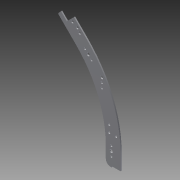
# Autodesk Inventor part: V5 Shooter Conveyor Plate P1 (45 Deg)
Saved by Autodesk Inventor 2014 SP1 (Build 180222100, 222)
## iProperties
Created: 2012-03-12
Part Number: V5 Shooter Conveyor Plate P1 (45 Deg)
Material: Aluminum-6061
Document SubType Name: Modeling
Designer: Moses
Mass: 110.618 g
Surface Area: 291.597 cm^2
Volume: 40.8185 cm^3
Density: 2.71 g/cm^3
Appearance: Aluminum - Flat
Author: Moses
Autodesk Inventor part; units mm, degrees
ref_plane "YZ Plane" through (0, 0, 0) normal (1, 0, 0) x (0, 1, 0)
ref_plane "XZ Plane" through (0, 0, 0) normal (0, 1, 0) x (-1, 0, 0)
ref_plane "XY Plane" through (0, 0, 0) normal (0, 0, 1) x (1, 0, 0)
sketch "Sketch1" plane through (0, 0, 0) normal (0, 0, 1) x (1, 0, 0)
  arc A0 (-15.749, 9.525) -> (-3.049, -3.175) centre (-3.049, 9.525) ccw
  line L0 (-3.049, -3.175) -> (0, -3.175)
  line L1 (0, -3.175) -> (0, 0)
  line L2 (0, 0) -> (24.5753, 0)
  line L3 (24.5753, 0) -> (24.5753, 41.4619)
  arc A1 (24.5753, 41.4619) -> (-69.0697, 267.5412) centre (-295.149, 41.4619) ccw
  line L4 (-69.0697, 267.5412) -> (-102.8779, 301.3493)
  line L5 (-102.8779, 301.3493) -> (-122.4112, 281.816)
  line L6 (-122.4112, 281.816) -> (-138.1267, 297.5314)
  line L7 (-138.1267, 297.5314) -> (-144.8619, 290.7962)
  arc A2 (-144.8619, 290.7962) -> (-144.8619, 286.3061) centre (-142.6168, 288.5511) ccw
  line L8 (-144.8619, 286.3061) -> (-97.5834, 239.0276)
  arc A3 (-15.749, 41.4619) -> (-97.5834, 239.0276) centre (-295.149, 41.4619) ccw
  line L9 (-15.749, 41.4619) -> (-15.749, 9.525)
  circle A4 centre (-1.0086, 22.225) radius 2.8448
  circle A5 centre (-1.0086, 47.625) radius 2.8448
  circle A6 centre (-26.9212, 171.2375) radius 2.85
  circle A7 centre (-26.9212, 183.9375) radius 2.85
  circle A8 centre (-26.9212, 196.6375) radius 4
  circle A9 centre (-73.0746, 241.3501) radius 2.85
  circle A10 centre (-55.1141, 223.3895) radius 2.85
  circle A11 centre (-7.1747, 76.2) radius 3.3782
  circle A12 centre (11.8753, 76.2) radius 3.3782
  circle A13 centre (-7.1747, 95.25) radius 3.3782
  circle A14 centre (-107.368, 287.8789) radius 3.3782
  circle A15 centre (-94.108, 280.5097) radius 3.3782
  circle A16 centre (-87.758, 270.9847) radius 3.3782
  circle A17 centre (-1.0086, 34.925) radius 4.15
  circle A18 centre (-64.0943, 232.3698) radius 4.15
  line L10 (-97.5834, 239.0276) -> (-69.0697, 267.5412) construction
  line L11 (-15.749, 41.4619) -> (24.5753, 41.4619) construction
  line L12 (-1.0086, 47.625) -> (-1.0086, 22.225) construction
  line L13 (-7.1747, 76.2) -> (11.8753, 76.2) construction
  line L14 (-7.1747, 76.2) -> (-7.1747, 95.25) construction
  line L15 (-26.9212, 196.6375) -> (-26.9212, 171.2375) construction
  line L16 (-73.0746, 241.3501) -> (-55.1141, 223.3895) construction
  dimension "d0" = 279.4
  dimension "d1" = 319.7243
  dimension "d2" = 6.7564
  dimension "d3" = 6.7564
  dimension "d4" = 6.7564
  dimension "d5" = 5.7
  dimension "d6" = 8.3
  dimension "d7" = 5.7
  dimension "d8" = 8
  dimension "d9" = 5.7
  dimension "d10" = 5.7
  dimension "d11" = 3.175
  dimension "d12" = 12.7
  dimension "d13" = 22.225
  dimension "d14" = 27.6243
  dimension "d15" = 47.8119
  dimension "d16" = 70.0369
  dimension "d17" = 66.8619
  dimension "d18" = 45
  dimension "d19" = 6.7564
  dimension "d20" = 6.7564
  dimension "d21" = 6.7564
  dimension "d22" = 5.6896
  dimension "d23" = 8.3
  dimension "d24" = 5.6896
  dimension "d25" = 12.7
  dimension "d26" = 3.049
  dimension "d27" = 24.5753
  dimension "d28" = 3.175
  dimension "d29" = 41.4619
  dimension "d30" = 31.9369
  dimension "d32" = 14.7404
  dimension "d33" = 22.225
  dimension "d34" = 34.7381
  dimension "d35" = 19.05
  dimension "d36" = 19.05
  dimension "d37" = 8.5743
  dimension "d38" = 11.1722
  dimension "d39" = 171.2375
  dimension "d40" = 18.9726
  dimension "d41" = 63.5
  dimension "d42" = 6.35
  dimension "d43" = 12.7
  dimension "d44" = 8.5346
  dimension "d46" = 20.9371
  dimension "d48" = 25.4
  dimension "d49" = 25.4
  dimension "d50" = 25.4
  dimension "d53" = 6.35
  dimension "d54" = 9.525
  constraints: 34 end point, 19 centre point, 8 point on circle, 7 perpendicular, 5 coincident, 5 parallel, 3 midpoint, 3 tangent, 1 vertical
  measures "d0" radius of A3
  measures "d1" radius of A1
  measures "d2" diameter of A14
  measures "d3" diameter of A15
  measures "d4" diameter of A16
  measures "d5" diameter of A9
  measures "d6" diameter of A18
  measures "d7" diameter of A10
  measures "d8" diameter of A8
  measures "d9" diameter of A7
  measures "d10" diameter of A6
  measures "d11" radius of A2
  measures "d12" distance between parallel lines of L6 L8
  measures "d13" distance of L5.end L6.end
  measures "d14" distance of L4.end L5.end
  measures "d15" distance of L4.start L4.end
  measures "d16" distance from line of L8.end L7
  measures "d17" distance of L8.start L8.end
  measures "d18" angle of L11 L10
  measures "d19" diameter of A13
  measures "d20" diameter of A11
  measures "d21" diameter of A12
  measures "d22" diameter of A5
  measures "d23" diameter of A17
  measures "d24" diameter of A4
  measures "d25" radius of A0
  measures "d26" distance of L0.start L0.end
  measures "d27" distance of L1.end L2.end
  measures "d28" distance of L0.end L1.end
  measures "d29" distance of L2.end L3.end
  measures "d30" distance of L9.start L9.end
  measures "d32" distance between parallel lines of L12 L9
  measures "d33" distance from line of L2 L12.end
  measures "d34" distance from line of L11 L13.start
  measures "d35" distance of L13.start L14.end
  measures "d36" distance of L13.start L13.end
  measures "d37" distance between parallel lines of L9 L14
  measures "d38" distance between parallel lines of L9 L15
  measures "d39" distance from line of L2 L15.end
  measures "d40" distance between parallel lines of L8 L16
  measures "d41" distance from line of L5 L16.start
  measures "d42" distance from line of L5 A14.centre
  measures "d43" distance from line of L4 A14.centre
  measures "d44" distance from line of L4 A15.centre
  measures "d46" distance from line of A15.centre L5
  measures "d48" distance of L12.start L12.end
  measures "d49" distance of L15.start L15.end
  measures "d50" distance of L16.start L16.end
  measures "d53" horizontal distance of A16.centre A15.centre
  measures "d54" vertical distance of A16.centre A15.centre
extrude "Extrusion1" add sketch "Sketch1" along normal blind 3.175
body "Solid1"
